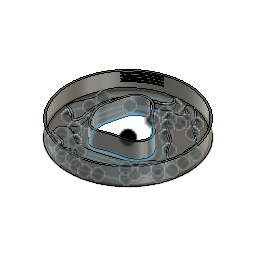
TreeCircleOrgan (Autodesk Fusion 360 design; units mm, degrees)
part number: 2026-04-19-12-51-08-975
part number: 2026-04-20-17-55-25-884
Autodesk Fusion 360 part; units mm, degrees
sketch "Sketch1" plane through (0, 0, 0) normal (0, 0, 1) x (1, 0, 0)
  circle A0 centre (0, 0) radius 49.5
  circle A1 centre (0, 0) radius 51
  spline S0 degree 5 poles (-2.5351, 23.5642) (-2.0298, 23.3804) (-1.0402, 22.9591) (0.3717, 22.1746) (2.087, 20.8696) (3.9595, 18.9553) (5.6153, 16.9147) (7.1415, 14.8871) (8.6424, 12.9685) (10.224, 11.1865) (11.9746, 9.5164) (13.9448, 7.8986) (16.1282, 6.2554) (18.4392, 4.5081) (20.7009, 2.5927) (22.6922, 0.4681) (24.1866, -1.8752) (24.995, -4.4062) (25.005, -7.0453) (24.2272, -9.6527) (22.7643, -12.0623) (20.773, -14.1185) (18.4282, -15.7141) (15.8872, -16.8251) (13.2509, -17.5525) (10.5751, -18.0743) (7.8852, -18.5901) (5.1907, -19.2663) (2.4982, -20.1876) (-0.1717, -21.2884) (-2.7841, -22.3736) (-5.2998, -23.1926) (-7.6815, -23.4995) (-9.9017, -23.1127) (-11.9516, -21.9909) (-13.8393, -20.2332) (-15.5765, -18.0166) (-17.1688, -15.5494) (-18.6058, -13.0228) (-19.847, -10.5524) (-20.8315, -8.1762) (-21.4994, -5.8814) (-21.8115, -3.6224) (-21.7667, -1.3426) (-21.4265, 1.0046) (-20.8923, 3.4492) (-20.2712, 6.0014) (-19.6445, 8.6488) (-19.0371, 11.3523) (-18.3824, 14.0425) (-17.5603, 16.6284) (-16.4359, 19.0059) (-14.8998, 21.0673) (-12.9053, 22.7095) (-10.5131, 23.8435) (-7.8618, 24.4029) (-5.6733, 24.3631) (-4.0722, 24.0619) (-3.0405, 23.748) (-2.5351, 23.5642) knots 0 0 0 0 0 0 0.018182 0.036364 0.054545 0.072727 0.090909 0.109091 0.127273 0.145455 0.163636 0.181818 0.2 0.218182 0.236364 0.254545 0.272727 0.290909 0.309091 0.327273 0.345455 0.363636 0.381818 0.4 0.418182 0.436364 0.454545 0.472727 0.490909 0.509091 0.527273 0.545455 0.563636 0.581818 0.6 0.618182 0.636364 0.654545 0.672727 0.690909 0.709091 0.727273 0.745455 0.763636 0.781818 0.8 0.818182 0.836364 0.854545 0.872727 0.890909 0.909091 0.927273 0.945455 0.963636 0.981818 1 1 1 1 1 1
  spline S1 degree 5 poles (-3.7406, 43.4351) (-2.9733, 43.1897) (-1.6249, 42.5335) (-0.2014, 41.1064) (0.3948, 38.6561) (-0.955, 35.6688) (-3.9837, 33.4865) (-7.827, 31.98) (-11.9429, 30.8133) (-15.9649, 29.5295) (-19.6815, 27.6641) (-22.9698, 24.8522) (-25.7494, 20.9363) (-27.9252, 16.0826) (-29.4137, 10.6775) (-30.1737, 5.2052) (-30.2329, 0.1449) (-29.7247, -4.1667) (-28.8996, -7.5981) (-28.2023, -10.4629) (-28.1356, -13.2049) (-29.0568, -15.9515) (-30.7596, -17.4477) (-32.6402, -15.6357) (-35.3107, -12.431) (-39.0161, -9.8567) (-43.3368, -9.2131) (-45.4002, -7.5209) (-44.7757, -4.0168) (-42.3903, 0.8003) (-39.7901, 5.8125) (-38.374, 9.9337) (-38.4705, 12.9017) (-39.4423, 15.1935) (-40.2444, 17.5576) (-39.8002, 20.7021) (-37.5307, 24.8444) (-33.39, 29.722) (-27.7054, 34.7855) (-21.0804, 39.334) (-14.2742, 42.6731) (-9.3274, 43.9444) (-6.2285, 44.006) (-4.5078, 43.6806) (-3.7406, 43.4351) knots 0 0 0 0 0 0 0.025 0.05 0.075 0.1 0.125 0.15 0.175 0.2 0.225 0.25 0.275 0.3 0.325 0.35 0.375 0.4 0.425 0.45 0.475 0.5 0.525 0.55 0.575 0.6 0.625 0.65 0.675 0.7 0.725 0.75 0.775 0.8 0.825 0.85 0.875 0.9 0.925 0.95 0.975 1 1 1 1 1 1
  line L0 (-32.81, -12.3441) -> (-49.7491, -6.6977)
  line L1 (-25.9956, -12.303) -> (-33.2624, -19.9422)
  spline S2 degree 3 poles (-0.826, 28.2631) (1.7075, 27.3415) (3.916, 25.8441) (5.6913, 24.2226) (7.6762, 22.4097) (9.1606, 20.4778) (10.4151, 18.8491) (11.6488, 17.2474) (12.6557, 15.9512) (13.7493, 14.8055) (14.8391, 13.6636) (16.0569, 12.6175) (17.64, 11.3912) (19.2697, 10.1287) (21.2908, 8.6958) (23.3418, 6.8482) (25.0705, 5.2909) (26.8163, 3.4232) (28.0943, 1.0851) (29.0918, -0.7398) (29.7684, -2.8718) (29.8826, -5.0619) (30.0133, -7.5696) (29.4169, -10.0756) (28.3339, -12.2532) (26.891, -15.1543) (24.6176, -17.5213) (22.0704, -19.1986) (19.8607, -20.6536) (17.46, -21.5595) (15.2782, -22.1424) (13.0567, -22.7358) (11.0763, -23.0486) (9.3068, -23.4354) (7.4518, -23.8409) (5.7916, -24.3288) (3.955, -25.0279) (2.2664, -25.6707) (0.4449, -26.4968) (-1.6304, -27.2112) (-3.3077, -27.7886) (-5.183, -28.2946) (-7.2633, -28.3274) (-8.9808, -28.3545) (-10.8128, -28.0035) (-12.4281, -27.2848) (-14.3816, -26.4156) (-15.9807, -25.0996) (-17.3079, -23.6904) (-19.1157, -21.7707) (-20.5047, -19.6531) (-21.7379, -17.5723) (-23.1703, -15.1552) (-24.3939, -12.7765) (-25.3177, -10.2757) (-26.0669, -8.2475) (-26.5832, -6.0914) (-26.7136, -3.9203) (-26.8489, -1.6698) (-26.5763, 0.5069) (-26.1861, 2.5196) (-25.735, 4.8458) (-25.1689, 7.0038) (-24.6447, 9.2527) (-24.1709, 11.2851) (-23.7274, 13.4278) (-23.0459, 15.7426) (-22.431, 17.8314) (-21.594, 20.0714) (-20.1946, 22.1718) (-18.9087, 24.1018) (-17.1226, 25.8598) (-15.0086, 27.0944) (-12.0537, 28.8202) (-8.5264, 29.5494) (-5.1155, 29.2296) (-3.6446, 29.0917) (-2.1946, 28.7609) (-0.826, 28.2631) knots 0 0 0 0 0.03910144 0.03910144 0.03910144 0.08281981 0.08281981 0.08281981 0.12581461 0.12581461 0.12581461 0.16866309 0.16866309 0.16866309 0.21277343 0.21277343 0.21277343 0.24995164 0.24995164 0.24995164 0.27897015 0.27897015 0.27897015 0.31219691 0.31219691 0.31219691 0.35646571 0.35646571 0.35646571 0.39486718 0.39486718 0.39486718 0.43396559 0.43396559 0.43396559 0.47495292 0.47495292 0.47495292 0.51264012 0.51264012 0.51264012 0.54310011 0.54310011 0.54310011 0.5682487 0.5682487 0.5682487 0.59866293 0.59866293 0.59866293 0.64009235 0.64009235 0.64009235 0.68821781 0.68821781 0.68821781 0.72724837 0.72724837 0.72724837 0.76770579 0.76770579 0.76770579 0.81446402 0.81446402 0.81446402 0.8567234 0.8567234 0.8567234 0.89485798 0.89485798 0.89485798 0.92989857 0.92989857 0.92989857 0.97887849 0.97887849 0.97887849 1 1 1 1
  spline S3 degree 5 poles (-2.5351, 23.5642) (-2.0298, 23.3804) (-1.0402, 22.9591) (0.3717, 22.1746) (2.087, 20.8696) (3.9595, 18.9553) (5.6153, 16.9147) (7.1415, 14.8871) (8.6424, 12.9685) (10.224, 11.1865) (11.9746, 9.5164) (13.9448, 7.8986) (16.1282, 6.2554) (18.4392, 4.5081) (20.7009, 2.5927) (22.6922, 0.4681) (24.1866, -1.8752) (24.995, -4.4062) (25.005, -7.0453) (24.2272, -9.6527) (22.7643, -12.0623) (20.773, -14.1185) (18.4282, -15.7141) (15.8872, -16.8251) (13.2509, -17.5525) (10.5751, -18.0743) (7.8852, -18.5901) (5.1907, -19.2663) (2.4982, -20.1876) (-0.1717, -21.2884) (-2.7841, -22.3736) (-5.2998, -23.1926) (-7.6815, -23.4995) (-9.9017, -23.1127) (-11.9516, -21.9909) (-13.8393, -20.2332) (-15.5765, -18.0166) (-17.1688, -15.5494) (-18.6058, -13.0228) (-19.847, -10.5524) (-20.8315, -8.1762) (-21.4994, -5.8814) (-21.8115, -3.6224) (-21.7667, -1.3426) (-21.4265, 1.0046) (-20.8923, 3.4492) (-20.2712, 6.0014) (-19.6445, 8.6488) (-19.0371, 11.3523) (-18.3824, 14.0425) (-17.5603, 16.6284) (-16.4359, 19.0059) (-14.8998, 21.0673) (-12.9053, 22.7095) (-10.5131, 23.8435) (-7.8618, 24.4029) (-5.6733, 24.3631) (-4.0722, 24.0619) (-3.0405, 23.748) (-2.5351, 23.5642) knots 0 0 0 0 0 0 0.018182 0.036364 0.054545 0.072727 0.090909 0.109091 0.127273 0.145455 0.163636 0.181818 0.2 0.218182 0.236364 0.254545 0.272727 0.290909 0.309091 0.327273 0.345455 0.363636 0.381818 0.4 0.418182 0.436364 0.454545 0.472727 0.490909 0.509091 0.527273 0.545455 0.563636 0.581818 0.6 0.618182 0.636364 0.654545 0.672727 0.690909 0.709091 0.727273 0.745455 0.763636 0.781818 0.8 0.818182 0.836364 0.854545 0.872727 0.890909 0.909091 0.927273 0.945455 0.963636 0.981818 1 1 1 1 1 1
  spline S4 degree 3 poles (-3.0479, 22.1546) (-0.8699, 21.3624) (1.034, 19.8482) (2.6858, 18.0359) (4.4056, 16.149) (5.869, 14.0027) (7.5057, 12.0473) (8.9313, 10.3439) (10.5243, 8.7791) (12.3565, 7.2854) (14.1883, 5.7919) (16.2751, 4.333) (18.1893, 2.7171) (20.0503, 1.1462) (21.6805, -0.5802) (22.5701, -2.3767) (23.5015, -4.2577) (23.6509, -6.2181) (23.0004, -8.1822) (22.3983, -10.0002) (21.1004, -11.7571) (19.4558, -13.0725) (17.8843, -14.3295) (16.0378, -15.1668) (14.0622, -15.7347) (11.9236, -16.3495) (9.601, -16.6888) (7.1996, -17.2474) (5.2068, -17.711) (3.165, -18.359) (1.2051, -19.1216) (-1.1812, -20.05) (-3.4558, -21.0885) (-5.3848, -21.5528) (-6.8661, -21.9093) (-8.0927, -21.9272) (-9.2253, -21.5611) (-10.3366, -21.202) (-11.4322, -20.4367) (-12.525, -19.2879) (-14.0527, -17.6818) (-15.5277, -15.3956) (-16.781, -13.156) (-17.9835, -11.0071) (-18.9691, -8.9223) (-19.5601, -7.0285) (-20.2391, -4.8526) (-20.3886, -2.8973) (-20.1203, -0.6773) (-19.8597, 1.4789) (-19.23, 3.9021) (-18.6146, 6.4999) (-18.0414, 8.9193) (-17.5178, 11.471) (-16.8473, 13.7809) (-16.1346, 16.2364) (-15.1865, 18.3739) (-13.7046, 19.9232) (-12.3938, 21.2936) (-10.6316, 22.2467) (-8.6515, 22.6226) (-6.8093, 22.9724) (-4.8352, 22.8047) (-3.0479, 22.1546) knots 0 0 0 0 0.053407 0.053407 0.053407 0.109014 0.109014 0.109014 0.157453 0.157453 0.157453 0.205884 0.205884 0.205884 0.252966 0.252966 0.252966 0.302262 0.302262 0.302262 0.347891 0.347891 0.347891 0.391491 0.391491 0.391491 0.438691 0.438691 0.438691 0.477859 0.477859 0.477859 0.525548 0.525548 0.525548 0.562171 0.562171 0.562171 0.598105 0.598105 0.598105 0.648342 0.648342 0.648342 0.696543 0.696543 0.696543 0.751923 0.751923 0.751923 0.805714 0.805714 0.805714 0.855811 0.855811 0.855811 0.909065 0.909065 0.909065 0.956172 0.956172 0.956172 1 1 1 1
  spline S5 degree 5 poles (-20.1069, -25.4022) (-20.5193, -25.1394) (-21.3713, -24.6344) (-22.7299, -23.9587) (-24.6686, -23.3072) (-27.1208, -23.1069) (-29.3679, -23.6604) (-31.1739, -25.0043) (-32.3466, -27.0332) (-32.7905, -29.446) (-32.4975, -31.8371) (-31.5288, -33.8119) (-30.0002, -35.0889) (-28.0661, -35.6173) (-25.9031, -35.6596) (-23.6886, -35.6292) (-21.5777, -35.9471) (-19.683, -36.9018) (-18.05, -38.4847) (-16.6435, -40.3032) (-15.3828, -41.8156) (-14.1709, -42.5297) (-12.9229, -42.1934) (-11.6017, -41.0453) (-10.2087, -39.6666) (-8.7602, -38.6968) (-7.2701, -38.6082) (-5.7259, -39.4209) (-4.1023, -40.8212) (-2.3807, -42.3473) (-0.564, -43.5379) (1.3004, -44.1265) (3.1234, -44.1133) (4.8235, -43.6422) (6.3612, -42.9267) (7.7871, -42.1477) (9.262, -41.3876) (10.9803, -40.6608) (13.1052, -39.9317) (15.7071, -39.1364) (18.6807, -38.2046) (21.7714, -37.0736) (24.6609, -35.6985) (27.0332, -34.0631) (28.6508, -32.1915) (29.4214, -30.157) (29.4821, -28.0977) (29.2348, -26.2137) (29.1699, -24.68) (29.7276, -23.578) (31.13, -22.8079) (33.2676, -22.0441) (35.8109, -20.9125) (38.2961, -19.1189) (40.2141, -16.6366) (41.1132, -13.7771) (40.65, -11.5557) (39.0766, -10.3515) (36.9208, -10.1655) (34.7819, -10.764) (33.0393, -11.8802) (31.7733, -13.3002) (30.883, -14.8491) (30.1508, -16.4029) (29.3317, -17.8907) (28.2227, -19.2985) (26.6655, -20.6481) (24.5547, -21.9795) (21.8447, -23.3315) (18.5565, -24.7238) (14.7849, -26.1377) (10.679, -27.525) (6.4209, -28.8174) (2.2053, -29.9358) (-1.7805, -30.7995) (-5.3775, -31.3354) (-8.4759, -31.4875) (-11.0342, -31.2256) (-13.1028, -30.5555) (-14.8365, -29.5264) (-16.4398, -28.2272) (-17.7835, -27.0718) (-18.8969, -26.2111) (-19.6945, -25.665) (-20.1069, -25.4022) knots 0 0 0 0 0 0 0.0125 0.025 0.0375 0.05 0.0625 0.075 0.0875 0.1 0.1125 0.125 0.1375 0.15 0.1625 0.175 0.1875 0.2 0.2125 0.225 0.2375 0.25 0.2625 0.275 0.2875 0.3 0.3125 0.325 0.3375 0.35 0.3625 0.375 0.3875 0.4 0.4125 0.425 0.4375 0.45 0.4625 0.475 0.4875 0.5 0.5125 0.525 0.5375 0.55 0.5625 0.575 0.5875 0.6 0.6125 0.625 0.6375 0.65 0.6625 0.675 0.6875 0.7 0.7125 0.725 0.7375 0.75 0.7625 0.775 0.7875 0.8 0.8125 0.825 0.8375 0.85 0.8625 0.875 0.8875 0.9 0.9125 0.925 0.9375 0.95 0.9625 0.975 0.9875 1 1 1 1 1 1
  line L2 (37.4302, -25.8713) -> (43.6842, -4.2949)
  spline S6 degree 5 poles (7.1051, 42.5099) (7.1257, 42.036) (7.2958, 41.0773) (7.9061, 39.7472) (9.2161, 38.6968) (11.1506, 38.1383) (12.8181, 37.5901) (13.7574, 36.319) (13.6773, 34.5327) (12.5114, 32.9542) (10.4313, 32.2665) (7.909, 32.4489) (5.6253, 32.7317) (4.1825, 32.345) (3.9357, 30.8624) (4.6165, 29.1689) (5.8847, 27.6074) (7.4096, 26.1869) (8.9194, 24.7545) (10.2803, 23.1836) (11.5266, 21.4939) (12.7835, 19.7731) (14.2056, 18.1329) (15.9159, 16.6568) (17.9284, 15.339) (20.1405, 14.0772) (22.3994, 12.7259) (24.5464, 11.1326) (26.4731, 9.1825) (28.1668, 6.8355) (29.776, 4.1765) (31.5463, 1.3949) (33.7015, -1.2531) (36.3765, -3.4815) (39.4546, -4.9996) (42.6145, -5.5689) (44.8894, -4.985) (45.4936, -3.2553) (44.745, -0.6762) (43.2891, 2.3526) (41.9402, 5.4155) (41.237, 8.2189) (41.1977, 10.6807) (41.5153, 12.8548) (41.7097, 14.876) (41.2979, 16.8955) (39.9508, 19.023) (37.6706, 21.2602) (34.7067, 23.5327) (31.4532, 25.7276) (28.3529, 27.7299) (25.7992, 29.4589) (24.038, 30.9049) (23.0714, 32.1653) (22.5541, 33.4834) (21.9631, 35.1362) (20.7854, 37.3052) (18.682, 39.9754) (15.7013, 42.7704) (12.3505, 44.9697) (9.333, 45.8229) (7.7223, 45.1513) (7.1722, 43.9204) (7.0845, 42.9838) (7.1051, 42.5099) knots 0 0 0 0 0 0 0.01666667 0.03333333 0.05 0.06666667 0.08333333 0.1 0.11666667 0.13333333 0.15 0.16666667 0.18333333 0.2 0.21666667 0.23333333 0.25 0.26666667 0.28333333 0.3 0.31666667 0.33333333 0.35 0.36666667 0.38333333 0.4 0.41666667 0.43333333 0.45 0.46666667 0.48333333 0.5 0.51666667 0.53333333 0.55 0.56666667 0.58333333 0.6 0.61666667 0.63333333 0.65 0.66666667 0.68333333 0.7 0.71666667 0.73333333 0.75 0.76666667 0.78333333 0.8 0.81666667 0.83333333 0.85 0.86666667 0.88333333 0.9 0.91666667 0.93333333 0.95 0.96666667 0.98333333 1 1 1 1 1 1
  line L3 (6.6913, 52.0261) -> (7.5188, 32.9937)
  line L4 (5.0364, 36.5795) -> (3.3088, 26.2727)
  line L5 (35.9294, -5.488) -> (49.1693, -5.0709)
  line L6 (4.4189, 40.1677) -> (-9.6109, 29.2176)
  point P0 (-2.596, 34.6926)
  point P1 (-23.0195, 24.3794)
  point P2 (-29.2868, -5.8569)
  point P3 (-29.629, -16.1226)
  point P4 (-41.2796, -9.5209)
  point P5 (-39.5487, 6.9036)
  point P6 (-39.9104, 18.6588)
  point P7 (-31.2078, -25.4022)
  point P8 (-30.1133, -34.7833)
  point P9 (-20.1069, -36.8158)
  point P10 (-13.8528, -42.2881)
  point P11 (-8.5369, -38.8484)
  point P12 (-1.2537, -43.0125)
  point P13 (6.0037, -43.0698)
  point P14 (14.0788, -39.6411)
  point P15 (29.1436, -30.5618)
  point P16 (29.769, -23.8387)
  point P17 (40.5572, -15.0831)
  point P18 (35.8667, -10.5489)
  point P19 (30.2381, -16.1775)
  point P20 (21.6388, -23.3696)
  point P21 (-10.5695, -31.1872)
  point P22 (12.8862, 37.2111)
  point P23 (11.3805, 32.7179)
  point P24 (4.1726, 31.4261)
  point P25 (8.4842, 25.1325)
  point P26 (15.1042, 17.4093)
  point P27 (26.827, 8.5827)
  point P28 (42.5494, -5.2795)
  point P29 (42.2735, 4.859)
  point P30 (40.9943, 17.0843)
  point P31 (24.1833, 30.9102)
  point P32 (19.1557, 39.2371)
  dimension "d25" = 99
  dimension "d26" = 1.5
  dimension "d27" = -5
  dimension "d28" = 0
  dimension "d29" = 1.5
  constraint coincident A0.centre A1.centre
  constraint midpoint P4 L0
  constraint midpoint P3 L1
  constraint midpoint P17 L2
  constraint midpoint S6.start L3
  constraint midpoint P24 L4
  constraint midpoint P28 L5
  constraint midpoint P0 L6
  measures "d25" diameter of A0
  measures "d28" distance of S0
  measures "d29" distance of S3
extrude "Extrude1" add sketch "Sketch1" along normal blind 14.5 contours A1 makes body 1
extrude "Extrude2" add sketch "Sketch1" along normal blind 1.5 contours A0 | S2 | L2 S6 L5 bodies 1
extrude "Extrude3" add sketch "Sketch1" along normal blind 6.5 contours S1 | S5 | S6 bodies 1
fillet "Fillet1" radius 1 3 faces at (-12.5358, 34.6302, 6.5) (28.1929, 21.4821, 6.5) (13.3624, -35.3934, 6.5) on bodies 1
sketch "Sketch2" plane through (0, 0, 6.5) normal (0, 0, 1) x (-1, 0, 0)
  spline S0 degree 3 poles (4.0452, -42.4827) (3.4062, -42.2783) (2.7926, -41.9742) (1.7986, -41.1208) (1.4171, -40.5763) (1.0565, -39.3649) (1.0727, -38.7149) (1.3514, -37.7633) (1.5065, -37.4274) (2.1719, -36.3411) (2.8561, -35.7147) (4.2841, -34.7148) (5.0255, -34.3195) (6.9307, -33.4472) (8.1222, -33.0296) (10.5224, -32.2538) (11.7327, -31.8975) (14.6916, -30.949) (16.4307, -30.3203) (19.9771, -28.4946) (21.7331, -27.2059) (24.9543, -23.821) (26.3257, -21.6621) (27.9791, -18.1885) (28.471, -16.9574) (29.6062, -13.6204) (30.1346, -11.4793) (30.807, -7.5469) (31.0035, -5.7566) (31.1436, -2.7036) (31.1457, -1.4484) (31.0287, 1.0439) (30.9098, 2.2761) (30.5994, 4.3827) (30.4343, 5.2681) (30.0834, 6.9194) (29.9024, 7.6849) (29.602, 9.0506) (29.4786, 9.6485) (29.3245, 10.7139) (29.2797, 11.1796) (29.2648, 12.0072) (29.2805, 12.3693) (29.3539, 12.9954) (29.3996, 13.2607) (29.5089, 13.7244) (29.5659, 13.924) (29.6848, 14.2703) (29.7426, 14.4183) (29.8543, 14.6681) (29.9051, 14.7715) (30.0096, 14.9627) (30.0623, 15.0509) (30.1561, 15.1908) (30.1946, 15.2442) (30.2813, 15.3546) (30.3301, 15.4109) (30.436, 15.5162) (30.4931, 15.566) (30.575, 15.617) (30.5939, 15.6275) (30.6333, 15.6454) (30.654, 15.6529) (30.6895, 15.6589) (30.7039, 15.6593) (30.7326, 15.6573) (30.7469, 15.655) (30.8066, 15.642) (30.8503, 15.6252) (30.9353, 15.5866) (30.9765, 15.5646) (31.1635, 15.4551) (31.2987, 15.3503) (31.5589, 15.1319) (31.6835, 15.0171) (32.184, 14.5369) (32.5448, 14.1495) (33.2731, 13.3878) (33.6383, 13.0118) (34.6716, 12.0118) (35.3633, 11.4117) (36.736, 10.4304) (37.3975, 10.033) (38.6161, 9.4327) (39.1626, 9.2057) (40.1425, 8.8455) (40.5718, 8.7028) (41.3375, 8.4474) (41.6739, 8.3352) (42.2212, 8.1274) (42.4355, 8.0394) (42.7909, 7.8659) (42.9352, 7.7872) (43.2676, 7.5681) (43.45, 7.4139) (43.6878, 7.0712) (43.7584, 6.8989) (43.8636, 6.4392) (43.8625, 6.1464) (43.8182, 5.6671) (43.7879, 5.4766) (43.645, 4.7665) (43.4844, 4.2592) (42.9282, 2.7218) (42.4625, 1.7145) (41.5099, -0.275) (41.0164, -1.2573) (40.025, -3.2849) (39.5259, -4.331) (38.8167, -6.0086) (38.5739, -6.6278) (38.0494, -8.1662) (37.7966, -9.0984) (37.5808, -10.6688) (37.5492, -11.2952) (37.6227, -12.5415) (37.7299, -13.1596) (38.0194, -14.2566) (38.1836, -14.7403) (38.5124, -15.706) (38.6758, -16.1895) (38.8523, -16.9704) (38.8993, -17.2587) (38.9936, -18.4041) (38.8517, -19.2671) (38.4421, -20.5522) (38.2562, -21.0077) (37.6076, -22.3847) (37.0688, -23.2679) (35.5149, -25.5177) (34.415, -26.8264) (32.09, -29.3136) (30.8607, -30.4911) (27.7806, -33.1973) (25.8797, -34.6732) (22.5732, -36.9391) (21.2094, -37.7949) (18.3483, -39.4079) (16.8476, -40.1607) (14.0957, -41.3207) (12.8617, -41.7679) (10.5895, -42.4035) (9.5604, -42.6264) (7.6962, -42.8538) (6.8651, -42.8949) (5.3632, -42.7966) (4.6898, -42.6888) (4.0452, -42.4827) knots 0 0 0 0 0.01232235 0.01232235 0.02405805 0.02405805 0.03553229 0.03553229 0.04226845 0.04226845 0.05892572 0.05892572 0.07428408 0.07428408 0.09742574 0.09742574 0.12056741 0.12056741 0.15455078 0.15455078 0.19397139 0.19397139 0.2403438 0.2403438 0.26465245 0.26465245 0.30505414 0.30505414 0.33817664 0.33817664 0.36107238 0.36107238 0.38385072 0.38385072 0.40059985 0.40059985 0.41502913 0.41502913 0.42612859 0.42612859 0.43466663 0.43466663 0.44133017 0.44133017 0.44626433 0.44626433 0.45005984 0.45005984 0.45297946 0.45297946 0.45510115 0.45510115 0.45698156 0.45698156 0.45818488 0.45818488 0.45955882 0.45955882 0.46093276 0.46093276 0.46133098 0.46133098 0.4617292 0.4617292 0.46199338 0.46199338 0.46225755 0.46225755 0.46311476 0.46311476 0.46397197 0.46397197 0.46709385 0.46709385 0.47021572 0.47021572 0.47983152 0.47983152 0.48944731 0.48944731 0.50634201 0.50634201 0.52046153 0.52046153 0.53132271 0.53132271 0.53960118 0.53960118 0.54612179 0.54612179 0.5503729 0.5503729 0.55338274 0.55338274 0.55768499 0.55768499 0.56104309 0.56104309 0.56634688 0.56634688 0.56988184 0.56988184 0.57964483 0.57964483 0.59990683 0.59990683 0.62016913 0.62016913 0.64142319 0.64142319 0.65364509 0.65364509 0.6713013 0.6713013 0.682757 0.682757 0.69421303 0.69421303 0.70359287 0.70359287 0.71297272 0.71297272 0.71832935 0.71832935 0.73407998 0.73407998 0.7430999 0.7430999 0.76204196 0.76204196 0.79331428 0.79331428 0.8245869 0.8245869 0.86867373 0.86867373 0.8982412 0.8982412 0.92901672 0.92901672 0.95308115 0.95308115 0.9723574 0.9723574 0.98757125 0.98757125 1 1 1 1
  circle A0 centre (8.6909, -12.5628) radius 35
  dimension "d39" = 70
  measures "d39" diameter of A0
extrude "Extrude4" cut sketch "Sketch2" along normal blind 1 contours S0 A0 picked at (10.2639, -9.8562) bodies 1
pattern_linear "R-Pattern1" count 5 spacing 2 along (0, 0, 1) of "Extrude4"
chamfer "Chamfer2" distance 0.3 angle 45 2 edges at (-28.6034, 41.3464, 7.5) (-28.6034, 41.3464, 9.5) on bodies 1
extrude "Extrude5" add sketch "Sketch1" along normal blind 14.5 contours S0 S3 bodies 1
copy_body "Body->Comp1" bodies 1 removing the originals makes body 2 in component "Circle Organ Top"
component "Circle Organ Top" placed x (1, 0, 0) y (0, 1, 0) z (0, 0, 1) at (0, 0, 0)
equation "WallThickness = 1.5 mm"
equation "ChamberHeight = 5 mm"
equation "InternalConnectionTubeThickness = 3 mm"
equation "InternalTubeFillet = 1 mm"
equation "ChamberFillet = 1 mm"
equation "TopSkinMaxThickness = 8 mm"
equation "BaseSkinMaxThickness = 8 mm"
equation "PipeHoleDiameter = 1.5 mm"
equation "TotalTopSkinHeigth = WallThickness + ChamberHeight + TopSkinMaxThickness"
equation "TotalBaseSkinHeigth = WallThickness + BaseSkinMaxThickness"
equation "Tolerances = 0.2 mm"
equation "OrganCoverExtraMargin = 10 mm"
equation "OrganCoverAdaperThickness = 2 mm"
equation "NumberOfToleranceDifferencesOrganCoverToHole = 4"
equation "OrganThicknessBelowCover = 4 mm"
equation "OrganFillet = 1 mm"
equation "CircleDiameter = 99 mm"
equation "d25 = CircleDiameter"
equation "d26 = WallThickness"
equation "d29 = WallThickness"
equation "d31 = TotalTopSkinHeigth"
equation "d33 = WallThickness"
equation "d35 = ChamberHeight + WallThickness"
equation "d38 = ChamberFillet"
equation "d48 = TotalTopSkinHeigth"
